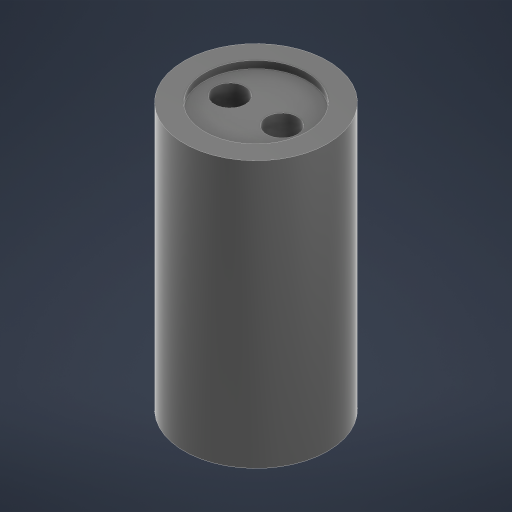
# Autodesk Inventor part: Abstandhalter_13mm
Saved by Autodesk Inventor 2023 (Build 270158000, 158)
## iProperties
Created: 2022-12-23
Part Number: Abstandhalter_13mm
Material: PC/ABS-Kunststoff
Document SubType Name: Modeling
Designer: Manuel
Density: 0.357273 g/cm^3
Appearance: Glatt - Schwarz
Author: Manuel
Autodesk Inventor part; units mm, degrees
ref_plane "YZ Plane" through (0, 0, 0) normal (1, 0, 0) x (0, 1, 0)
ref_plane "XZ Plane" through (0, 0, 0) normal (0, 1, 0) x (-1, 0, 0)
ref_plane "XY Plane" through (0, 0, 0) normal (0, 0, 1) x (1, 0, 0)
sketch "Skizze1" plane through (0, 0, 0) normal (0, 1, 0) x (-1, 0, 0)
  circle A0 centre (0, 0) radius 3.5
  dimension "d0" = 7
  constraints: 1 centre point, 1 coincident
  measures "d0" diameter of A0
extrude "Extrusion1" add sketch "Skizze1" along normal blind 13
sketch "Skizze2" plane through (0, 13, 0) normal (0, 1, 0) x (1, 0, 0)
  circle A0 centre (0, 0) radius 2.5
  dimension "d3" = 5
  constraints: 1 centre point, 1 coincident
  measures "d3" diameter of A0
extrude "Extrusion2" cut sketch "Skizze2" against normal blind 0.35
sketch "Skizze3" plane through (0, 12.65, 0) normal (0, 1, 0) x (1, 0, 0)
  line L0 (0, 0) -> (0, 2.5) construction
  circle A0 centre (0, 0) radius 2.5 construction
  circle A1 centre (-1.27, 0) radius 0.75
  circle A2 centre (1.27, 0) radius 0.75
  dimension "d6" = 1.5
  dimension "d7" = 2.54
  constraints: 2 centre point, 2 end point, 1 horizontal alignment, 1 symmetric about line, 1 vertical, 1 vertical alignment, 2 other
  measures "d6" diameter of A1
  measures "d7" distance of A2.centre A1.centre
extrude "Extrusion3" cut sketch "Skizze3" against normal through all
